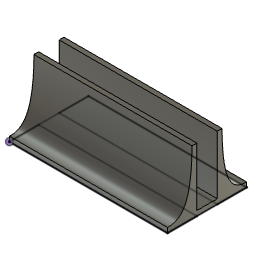
mac_rack (Autodesk Fusion 360 design; units mm, degrees)
Autodesk Fusion 360 part; units mm, degrees
sketch "Sketch1" plane through (0, 0, 0) normal (0, 0, 1) x (1, 0, 0)
  line L0 (0, 0) -> (100, 0)
  line L1 (100, 0) -> (100, 50)
  line L2 (100, 50) -> (0, 50)
  line L3 (0, 50) -> (0, 0)
  line L4 (0, 0) -> (100, 0)
  line L5 (100, 0) -> (100, 18.5)
  line L6 (100, 18.5) -> (0, 18.5)
  line L7 (0, 18.5) -> (0, 0)
  line L8 (0, 50) -> (100, 50)
  line L9 (100, 50) -> (100, 31.5)
  line L10 (100, 31.5) -> (0, 31.5)
  line L11 (0, 31.5) -> (0, 50)
  dimension "d1" = 100
  dimension "d2" = 50
  dimension "d3" = 18.5
  dimension "d4" = 18.5
  constraint horizontal L0
  constraint vertical L1
  constraint horizontal L2
  constraint vertical L3
  constraint coincident L0.start L3.end
  constraint horizontal L4
  constraint vertical L5
  constraint horizontal L6
  constraint vertical L7
  constraint coincident L1 L5.end
  constraint horizontal L8
  constraint vertical L9
  constraint horizontal L10
  constraint vertical L11
  constraint coincident L1 L9.end
  measures "d1" distance of L0.start L0.end
  measures "d2" distance of L0.start L2.end
  measures "d3" distance of L0.start L6.end
  measures "d4" distance of L2.end L10.end
extrude "Extrude1" add sketch "Sketch1" along normal blind 3 contours L1 L3 L6 L10
extrude "Extrude2" add sketch "Sketch1" along normal blind 40 contours L0 L1 L3 L4 L5 L6 L7 | L1 L2 L3 L8 L9 L10 L11
sketch "Sketch2" plane through (100, 0, 0) normal (1, 0, 0) x (0, 1, 0)
  line L0 (0, 0) -> (50, 0)
  line L1 (50, 0) -> (50, 40)
  line L2 (50, 40) -> (31.5, 40)
  line L3 (31.5, 40) -> (31.5, 3)
  line L4 (31.5, 3) -> (18.5, 3)
  line L5 (18.5, 3) -> (18.5, 40)
  line L6 (18.5, 40) -> (0, 40)
  line L7 (0, 40) -> (0, 0)
  line L8 (18.5, 40) -> (15.5, 40)
  line L9 (31.5, 40) -> (34.5, 40)
  spline S0 degree 5 poles (0, 3) (0.6686, 2.9687) (1.9704, 2.982) (3.8176, 3.2291) (6.0657, 4.0208) (8.4986, 5.8217) (10.5348, 8.4758) (12.1729, 11.9864) (13.442, 16.2906) (14.3808, 21.3051) (15.0282, 26.9468) (15.3373, 31.909) (15.4603, 35.8649) (15.4947, 38.6046) (15.5, 40) knots 0 0 0 0 0 0 0.1 0.2 0.3 0.4 0.5 0.6 0.7 0.8 0.9 1 1 1 1 1 1
  spline S1 degree 5 poles (50, 3) (49.3314, 2.9687) (48.0296, 2.982) (46.1824, 3.2291) (43.9343, 4.0208) (41.5014, 5.8217) (39.4652, 8.4758) (37.8271, 11.9864) (36.558, 16.2906) (35.6192, 21.3051) (34.9718, 26.9468) (34.6627, 31.909) (34.5397, 35.8649) (34.5053, 38.6046) (34.5, 40) knots 0 0 0 0 0 0 0.1 0.2 0.3 0.4 0.5 0.6 0.7 0.8 0.9 1 1 1 1 1 1
  line L10 (34.5, 40) -> (50, 40)
  line L11 (50, 3) -> (50, 40)
  line L12 (0, 3) -> (0, 40)
  line L13 (15.5, 40) -> (0, 40)
  point P0 (10, 8)
  point P1 (40, 8)
  dimension "d9" = 3
  dimension "d10" = 3
  constraint coincident L5.end L6.start
  constraint perpendicular L5 L8
  constraint coincident L2.end L3.start
  constraint perpendicular L3 L9
  constraint coincident L7 S0.start
  constraint coincident L1 S1.start
  constraint coincident L1.end L2.start
  constraint coincident L6.end L7.start
  constraint perpendicular L6 L12
  measures "d9" distance of L5.end L8.end
  measures "d10" distance of L2.end L9.end
extrude "Extrude3" cut sketch "Sketch2" against normal blind 100 contours L6 L7 S0 L12 L13 | L1 L2 S1 L10 L11
